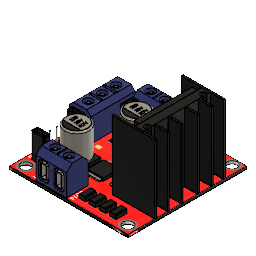
l298n (Autodesk Fusion 360 design; units mm, degrees)
Autodesk Fusion 360 part; units mm, degrees
note: some values were not read from the file. Chosen so that the rebuilt part matches the saved one: which face or edge a step refers to. Set by a fixed rule: which sketch regions a step uses.
(part 1 of 2)
sketch "Sketch2" plane through (0, 0, 0) normal (0, 1, 0) x (1, 0, 0)
  line L0 (-21.58, 21.58) -> (21.58, 21.58)
  line L1 (21.58, 21.58) -> (21.58, -21.58)
  line L2 (21.58, -21.58) -> (-21.58, -21.58)
  line L3 (-21.58, -21.58) -> (-21.58, 21.58)
  dimension "d1" = 43.16
  dimension "d2" = 43.16
extrude "Extrude1" add sketch "Sketch2" along normal blind 1 makes body 1
sketch "Sketch3" plane through (0, 1, 0) normal (0, 1, 0) x (-1, 0, 0)
  line L0 (21.58, 21.58) -> (-21.58, 21.58)
  line L1 (-21.58, 21.58) -> (-21.58, -21.58)
  line L2 (-21.58, -21.58) -> (21.58, -21.58)
  line L3 (21.58, -21.58) -> (21.58, 21.58)
  circle A0 centre (18.5683, 18.5343) radius 1.8
  circle A1 centre (-18.5859, 18.5894) radius 1.8
  circle A2 centre (18.6014, -19.35) radius 1.8
  circle A3 centre (-18.5529, -19.2949) radius 1.8
  line L4 (15.2987, 12.0305) -> (6.6207, 12.0305)
  line L5 (6.6207, 12.0305) -> (6.6207, 3.2285)
  line L6 (6.6207, 3.2285) -> (15.2987, 3.2285)
  line L7 (15.2987, 3.2285) -> (15.2987, 12.0305)
  line L8 (15.2987, 4.5307) -> (14.0438, 3.2285)
  dimension "d5" = 3.6
  dimension "d6" = 3.6
  dimension "d7" = 3.6
  dimension "d8" = 3.6
  dimension "d13" = 37.1543
  dimension "d14" = 37.1543
  measures "d5" diameter of A0
  measures "d6" diameter of A1
  measures "d7" diameter of A2
  measures "d8" diameter of A3
extrude "Extrude2" cut sketch "Sketch3" along normal blind 3 and the other way blind 2 contours A0 | A1 | A2 | A3 bodies 1
sketch "Sketch4" plane through (0, 1, 0) normal (0, 1, 0) x (-1, 0, 0)
  circle A0 centre (-18.5529, -19.2949) radius 1.8
  circle A1 centre (18.6014, -19.35) radius 1.8
  circle A2 centre (-18.5859, 18.5894) radius 1.8
  circle A3 centre (18.5683, 18.5343) radius 1.8
  line L0 (21.58, 21.58) -> (-21.58, 21.58)
  line L1 (-21.58, 21.58) -> (-21.58, -21.58)
  line L2 (-21.58, -21.58) -> (21.58, -21.58)
  line L3 (21.58, -21.58) -> (21.58, 21.58)
  line L4 (-8.5487, -11.3714) -> (-11.814, -11.3714)
  line L5 (-11.814, -11.3714) -> (-11.814, 9.6641)
  line L6 (-11.814, 9.6641) -> (-8.5487, 9.6641)
  line L7 (-8.1487, 9.2641) -> (-8.1487, -10.9714)
  arc A4 (-8.5487, -11.3714) -> (-8.1487, -10.9714) centre (-8.5487, -10.9714) ccw
  arc A5 (-8.1487, 9.2641) -> (-8.5487, 9.6641) centre (-8.5487, 9.2641) ccw
  line L8 (-13.7341, -13.1256) -> (-16.7801, -13.1256)
  line L9 (-16.7801, -13.1256) -> (-16.7801, 11.2965)
  line L10 (-16.7801, 11.2965) -> (-13.7341, 11.2965)
  line L11 (-13.7341, 11.2965) -> (-13.7341, -13.1256)
  dimension "d15" = 0.4
  dimension "d16" = 0.4
  measures "d15" radius of A4
  measures "d16" radius of A5
extrude "Extrude3" add sketch "Sketch4" along normal blind 15 contours L4 L5 L6 L7 A4 A5 bodies 1
delete_face "DeleteFace1" 7 faces at (8.2229, 11, -11.2034) (8.1487, 6, 2.5189) (8.1774, 11, 9.4127) (10.7256, 6, 9.6641) (11.814, 6, -4.3596) (9.6372, 6, -11.3714) (10.5923, 16, -4.2263) on bodies 1
sketch "Sketch5" plane through (0, 1, 0) normal (0, 1, 0) x (-1, 0, 0)
  circle A0 centre (-18.5529, -19.2949) radius 1.8
  circle A1 centre (18.6014, -19.35) radius 1.8
  circle A2 centre (-18.5859, 18.5894) radius 1.8
  circle A3 centre (18.5683, 18.5343) radius 1.8
  line L0 (-21.58, 21.58) -> (-21.58, -21.58)
  line L1 (-21.58, -21.58) -> (21.58, -21.58)
  line L2 (21.58, -21.58) -> (21.58, 21.58)
  line L3 (21.58, 21.58) -> (-21.58, 21.58)
  line L4 (-9.1628, -11.5053) -> (-11.8128, -11.5053)
  line L5 (-11.8128, -11.5053) -> (-11.8128, 9.6008)
  line L6 (-11.8128, 9.6008) -> (-9.1628, 9.6008)
  line L7 (-8.1628, 8.6008) -> (-8.1628, -10.5053)
  arc A4 (-9.1628, -11.5053) -> (-8.1628, -10.5053) centre (-9.1628, -10.5053) ccw
  arc A5 (-8.1628, 8.6008) -> (-9.1628, 9.6008) centre (-9.1628, 8.6008) ccw
  line L8 (-11.8128, -11.5053) -> (-13.7787, -11.5053)
  line L9 (-13.7787, -11.5053) -> (-13.7787, 9.5847)
  line L10 (-13.7787, 9.5847) -> (-11.8128, 9.5847)
  line L11 (-11.8128, 9.5847) -> (-11.8128, -11.5053)
  dimension "d19" = 1
  dimension "d20" = 1
  dimension "d25" = 3.65
  measures "d19" radius of A4
  measures "d20" radius of A5
  measures "d25" distance of L5 L7
extrude "Extrude8" add sketch "Sketch5" along normal blind 25 separate body contours L5 L8 L9 L10 L11 makes body 2
extrude "Extrude5" add sketch "Sketch5" along normal blind 15 separate body contours L4 L5 L6 L7 A4 A5 L11 makes body 3
sketch "Sketch6" plane through (11.8128, 0, 0) normal (1, 0, 0) x (0, 0, -1)
  line L0 (-9.6008, 1) -> (11.5053, 1)
  line L1 (11.5053, 1) -> (11.5053, 16)
  line L2 (11.5053, 16) -> (-9.6008, 16)
  line L3 (-9.6008, 16) -> (-9.6008, 1)
  circle A0 centre (-9.6008, 8.5) radius 2
  circle A1 centre (11.5053, 8.5) radius 2
  circle A2 centre (-4.6008, 8.5) radius 1
  circle A3 centre (6.5053, 8.5) radius 1
  dimension "d26" = 4
  dimension "d27" = 4
  dimension "d28" = 2
  dimension "d29" = 2
  measures "d26" diameter of A0
  measures "d27" diameter of A1
  measures "d28" diameter of A2
  measures "d29" diameter of A3
extrude "Extrude7" add sketch "Sketch6" against normal blind 4 contours A2 | A3 bodies 3
extrude "Extrude6" cut sketch "Sketch6" along normal blind 2 and the other way blind 6 contours L3 A0 | L3 A0 | L1 A1 | L1 A1 bodies 3
box "BoxPrimitive1" cut length 1.9835 width 0.2553 height -0.2 placed x (0, 1, 0) y (0, 0, -1) z (-1, 0, 0) at (7.8128, 7.5069, -6.3882) bodies 3
box "BoxPrimitive2" cut length 0.319 width 1.9733 height -0.2 placed x (0, 1, 0) y (0, 0, -1) z (-1, 0, 0) at (7.8128, 8.3724, -5.5135) bodies 3
box "BoxPrimitive3" cut length 1.9717 width 0.332 height -0.2 placed x (0, 1, 0) y (0, 0, -1) z (-1, 0, 0) at (7.8128, 7.5102, 4.7436) bodies 3
box "BoxPrimitive4" cut length 0.3057 width 1.9763 height -0.2 placed x (0, 1, 0) y (0, 0, -1) z (-1, 0, 0) at (7.8128, 8.3339, 5.587) bodies 3
box "BoxPrimitive5" add length 6.5992 width 21.1061 height 1.5 placed x (0, -1, 0) y (0, 0, 1) z (-1, 0, 0) at (11.8128, 22.5992, -11.5053) separate body makes body 4
chamfer "Chamfer1" distance 2 angle 45 1 edges at (11.0628, 22.5992, -11.5053) on bodies 4
chamfer "Chamfer2" distance 2 angle 45 1 edges at (11.0628, 22.5992, 9.6008) on bodies 4
sketch "Sketch12" plane through (10.3128, 0, 0) normal (-1, 0, 0) x (0, 0, 1)
  line L0 (9.6008, 20.5992) -> (7.6008, 22.5992)
  line L1 (7.6008, 22.5992) -> (-9.5053, 22.5992)
  line L2 (-9.5053, 22.5992) -> (-11.5053, 20.5992)
  line L3 (-11.5053, 20.5992) -> (-11.5053, 16)
  line L4 (9.6008, 16) -> (9.6008, 20.5992)
  circle A0 centre (-0.9522, 19.645) radius 1
  line L5 (-11.5053, 16) -> (9.6008, 16)
  dimension "d67" = 2
  measures "d67" diameter of A0
extrude "Extrude9" add sketch "Sketch12" along normal blind 0.5 separate body contours A0 makes body 5
box "BoxPrimitive6" cut length 1.5257 width 0.3014 height -0.5 placed x (0, 1, 0) y (0, 0, -1) z (-1, 0, 0) at (9.8128, 18.8541, -0.7916) bodies 5
box "BoxPrimitive7" cut length 0.2355 width 1.4127 height -0.5 placed x (0, 1, 0) y (0, 0, -1) z (-1, 0, 0) at (9.8128, 19.617, -0.2265) bodies 5
fillet "Fillet1" radius 0.2 1 edges at (9.8128, 19.2834, -1.8846) on bodies 5
box "BoxPrimitive8" add length 24.4221 width 3.046 height 25 placed x (0, 0, 1) y (1, 0, 0) z (0, 1, 0) at (13.7341, 1, -13.1256) separate body makes body 6
cylinder "CylinderPrimitive1" cut diameter 2 height -25 placed x (1, 0, 0) y (0, 0, -1) z (0, 1, 0) at (16.0686, 26, -11.2277) bodies 6
cylinder "CylinderPrimitive2" cut diameter 2 height -25 placed x (1, 0, 0) y (0, 0, -1) z (0, 1, 0) at (16.0862, 26, 9.0521) bodies 6
box "BoxPrimitive9" add length 0.6958 width 15.4001 height 25 placed x (0, 0, 1) y (1, 0, 0) z (0, 1, 0) at (6.1799, 1, 11.1734) separate body makes body 7
copy_body "CopyPasteBodies1" bodies 7 makes body 8
move_body "Move1" bodies 8 to x (1, 0, 0) y (0, 1, 0) z (0, 0, 1) at (0, 0, -25)
box "BoxPrimitive20" add length 0.9521 width 4.9337 height 0.5 placed x (0, 0, 1) y (1, 0, 0) z (0, 1, 0) at (-4.9818, 1, 9.3224) separate body makes body 9
box "BoxPrimitive10" add length 0.6636 width 4.7999 height 25 placed x (0, 0, -1) y (-1, 0, 0) z (0, 1, 0) at (21.58, 1, 7.2397) separate body makes body 10
copy_body "CopyPasteBodies2" bodies 10 makes body 11
move_body "Move2" bodies 11 to x (1, 0, 0) y (0, 1, 0) z (0, 0, 1) at (0, 0, -5)
copy_body "CopyPasteBodies3" bodies 11 makes body 12
move_body "Move3" bodies 12 to x (1, 0, 0) y (0, 1, 0) z (0, 0, 1) at (0, 0, -6)
copy_body "CopyPasteBodies4" bodies 12 makes body 13
move_body "Move4" bodies 13 to x (1, 0, 0) y (0, 1, 0) z (0, 0, 1) at (0, 0, -5)
box "BoxPrimitive11" add length 8.802 width 8.678 height 1 placed x (0, 0, 1) y (1, 0, 0) z (0, 1, 0) at (-15.2987, 1, 3.2285) separate body makes body 14
copy_body "CopyPasteBodies5" bodies 14 makes body 15
move_body "Move5" bodies 15 to x (1, 0, 0) y (0, 1, 0) z (0, 0, 1) at (7.2382, 0, -14.5913)
sketch "Sketch23" plane through (0, 2, 0) normal (0, 1, 0) x (-1, 0, 0)
  line L0 (15.2987, 12.0305) -> (6.6207, 12.0305)
  line L1 (6.6207, 12.0305) -> (6.6207, 3.2285)
  line L2 (6.6207, 3.2285) -> (15.2987, 3.2285)
  line L3 (15.2987, 3.2285) -> (15.2987, 12.0305)
  line L4 (15.2987, 3.2285) -> (6.6207, 12.0305) construction
  line L5 (6.6207, 3.2285) -> (15.2987, 12.0305) construction
cylinder "CylinderPrimitive3" add diameter 8.678 height 11 placed x (1, 0, 0) y (0, 0, -1) z (0, 1, 0) at (-10.9597, 2, 7.6295) separate body makes body 16
fillet "Fillet2" radius 1 1 edges at (-15.005, 2, 6.0605) on bodies 16
fillet "Fillet3" radius 0.5 1 edges at (-15.005, 13, 9.1986) on bodies 16
sketch "Sketch24" plane through (0, 13, 0) normal (0, 1, 0) x (-1, 0, 0)
  circle A0 centre (10.9597, 7.6295) radius 3.839
  line L0 (14.3816, 9.3698) -> (7.5378, 9.3698)
extrude "Extrude11" add sketch "Sketch24" along normal blind 0.1 contours A0 L0 picked at (9.791, 7.9606) bodies 16
extrude "Extrude10" add sketch "Sketch24" along normal blind 0.1 separate body contours A0 L0 picked at (10.272, 9.961) makes body 17
fillet "Fillet4" radius 0.1 1 edges at (-10.9597, 13.1, 11.4685) on bodies 17
fillet "Fillet5" radius 0.1 1 edges at (-10.9597, 13.1, 3.7905) on bodies 16
sketch "Sketch25" plane through (0, 13.1, 0) normal (0, 1, 0) x (-1, 0, 0)
  arc A0 (7.6504, 9.3698) -> (14.269, 9.3698) centre (10.9597, 7.6295) ccw
  line L0 (14.269, 9.3698) -> (7.6504, 9.3698)
  line L1 (12.3518, 7.4819) -> (12.1607, 7.4819)
  line L2 (12.1607, 7.4819) -> (12.1607, 8.2033)
  spline S0 degree 3 poles (12.1607, 8.2033) (12.1965, 8.1973) (12.2689, 8.1853) (12.3335, 8.1505) (12.3661, 8.133) knots 0 0 0 0 0.010813 0.021847 0.021847 0.021847 0.021847
  spline S1 degree 3 poles (12.3661, 8.133) (12.4046, 8.1049) (12.4981, 8.0365) (12.5771, 7.9515) (12.6236, 7.9015) knots 0 0 0 0 0.014262 0.034686 0.034686 0.034686 0.034686
  spline S2 degree 3 poles (12.6236, 7.9015) (12.6589, 7.8631) (12.7142, 7.8028) (12.7767, 7.75) (12.7993, 7.7309) knots 0 0 0 0 0.01563 0.024519 0.024519 0.024519 0.024519
  spline S3 degree 3 poles (12.7993, 7.7309) (12.8199, 7.7185) (12.8588, 7.695) (12.904, 7.6905) (12.9253, 7.6884) knots 0 0 0 0 0.007091 0.013443 0.013443 0.013443 0.013443
  spline S4 degree 3 poles (12.9253, 7.6884) (12.9464, 7.6894) (12.9855, 7.6913) (13.0167, 7.7146) (13.0312, 7.7254) knots 0 0 0 0 0.006158 0.01144 0.01144 0.01144 0.01144
  spline S5 degree 3 poles (13.0312, 7.7254) (13.0419, 7.7395) (13.0649, 7.7695) (13.067, 7.8074) (13.0681, 7.8276) knots 0 0 0 0 0.005205 0.011091 0.011091 0.011091 0.011091
  spline S6 degree 3 poles (13.0681, 7.8276) (13.0669, 7.8476) (13.0644, 7.8859) (13.0406, 7.9158) (13.0293, 7.9301) knots 0 0 0 0 0.005867 0.0112 0.0112 0.0112 0.0112
  spline S7 degree 3 poles (13.0293, 7.9301) (13.0126, 7.9415) (12.974, 7.9679) (12.9271, 7.9718) (12.9004, 7.974) knots 0 0 0 0 0.005973 0.013825 0.013825 0.013825 0.013825
  line L3 (12.9004, 7.974) -> (12.9209, 8.1791)
  spline S8 degree 3 poles (12.9209, 8.1791) (12.9721, 8.1715) (13.0655, 8.1577) (13.1339, 8.0933) (13.1648, 8.0641) knots 0 0 0 0 0.015078 0.027543 0.027543 0.027543 0.027543
  spline S9 degree 3 poles (13.1648, 8.0641) (13.1864, 8.0288) (13.2317, 7.9548) (13.2363, 7.8679) (13.2388, 7.8224) knots 0 0 0 0 0.01221 0.025631 0.025631 0.025631 0.025631
  spline S10 degree 3 poles (13.2388, 7.8224) (13.2363, 7.7735) (13.2316, 7.6817) (13.1781, 7.6074) (13.1531, 7.5727) knots 0 0 0 0 0.014351 0.026906 0.026906 0.026906 0.026906
  spline S11 degree 3 poles (13.1531, 7.5727) (13.1227, 7.5462) (13.0615, 7.4929) (12.9806, 7.4856) (12.94, 7.4819) knots 0 0 0 0 0.011782 0.0237 0.0237 0.0237 0.0237
  spline S12 degree 3 poles (12.94, 7.4819) (12.9162, 7.4829) (12.8689, 7.485) (12.8241, 7.5003) (12.8019, 7.5079) knots 0 0 0 0 0.007107 0.014113 0.014113 0.014113 0.014113
  spline S13 degree 3 poles (12.8019, 7.5079) (12.7791, 7.5183) (12.7303, 7.5408) (12.6874, 7.5731) (12.6646, 7.5903) knots 0 0 0 0 0.007505 0.016056 0.016056 0.016056 0.016056
  spline S14 degree 3 poles (12.6646, 7.5903) (12.645, 7.6074) (12.5967, 7.6497) (12.5534, 7.697) (12.5276, 7.725) knots 0 0 0 0 0.007818 0.019227 0.019227 0.019227 0.019227
  spline S15 degree 3 poles (12.5276, 7.725) (12.5032, 7.7519) (12.4647, 7.7941) (12.4238, 7.8339) (12.409, 7.8484) knots 0 0 0 0 0.010889 0.017123 0.017123 0.017123 0.017123
  spline S16 degree 3 poles (12.409, 7.8484) (12.3995, 7.8565) (12.3815, 7.872) (12.3614, 7.8846) (12.3518, 7.8905) knots 0 0 0 0 0.003729 0.007106 0.007106 0.007106 0.007106
  line L4 (12.3518, 7.8905) -> (12.3518, 7.4819)
  line L5 (12.3518, 6.6476) -> (12.1607, 6.6476)
  line L6 (12.1607, 6.6476) -> (12.1607, 7.3691)
  spline S17 degree 3 poles (12.1607, 7.3691) (12.1965, 7.3631) (12.2689, 7.3511) (12.3335, 7.3163) (12.3661, 7.2987) knots 0 0 0 0 0.010813 0.021847 0.021847 0.021847 0.021847
  spline S18 degree 3 poles (12.3661, 7.2987) (12.4046, 7.2706) (12.4981, 7.2022) (12.5771, 7.1173) (12.6236, 7.0673) knots 0 0 0 0 0.014262 0.034686 0.034686 0.034686 0.034686
  spline S19 degree 3 poles (12.6236, 7.0673) (12.6589, 7.0289) (12.7142, 6.9686) (12.7767, 6.9158) (12.7993, 6.8967) knots 0 0 0 0 0.01563 0.024519 0.024519 0.024519 0.024519
  spline S20 degree 3 poles (12.7993, 6.8967) (12.8199, 6.8843) (12.8588, 6.8608) (12.904, 6.8563) (12.9253, 6.8542) knots 0 0 0 0 0.007091 0.013443 0.013443 0.013443 0.013443
  spline S21 degree 3 poles (12.9253, 6.8542) (12.9464, 6.8552) (12.9855, 6.8571) (13.0167, 6.8804) (13.0312, 6.8912) knots 0 0 0 0 0.006158 0.01144 0.01144 0.01144 0.01144
  spline S22 degree 3 poles (13.0312, 6.8912) (13.0419, 6.9053) (13.0649, 6.9353) (13.067, 6.9732) (13.0681, 6.9933) knots 0 0 0 0 0.005205 0.011091 0.011091 0.011091 0.011091
  spline S23 degree 3 poles (13.0681, 6.9933) (13.0669, 7.0134) (13.0644, 7.0516) (13.0406, 7.0816) (13.0293, 7.0959) knots 0 0 0 0 0.005867 0.0112 0.0112 0.0112 0.0112
  spline S24 degree 3 poles (13.0293, 7.0959) (13.0126, 7.1073) (12.974, 7.1337) (12.9271, 7.1376) (12.9004, 7.1398) knots 0 0 0 0 0.005973 0.013825 0.013825 0.013825 0.013825
  line L7 (12.9004, 7.1398) -> (12.9209, 7.3449)
  spline S25 degree 3 poles (12.9209, 7.3449) (12.9721, 7.3373) (13.0655, 7.3235) (13.1339, 7.259) (13.1648, 7.2299) knots 0 0 0 0 0.015078 0.027543 0.027543 0.027543 0.027543
  spline S26 degree 3 poles (13.1648, 7.2299) (13.1864, 7.1946) (13.2317, 7.1205) (13.2363, 7.0337) (13.2388, 6.9882) knots 0 0 0 0 0.01221 0.025631 0.025631 0.025631 0.025631
  spline S27 degree 3 poles (13.2388, 6.9882) (13.2363, 6.9392) (13.2316, 6.8475) (13.1781, 6.7731) (13.1531, 6.7384) knots 0 0 0 0 0.014351 0.026906 0.026906 0.026906 0.026906
  spline S28 degree 3 poles (13.1531, 6.7384) (13.1227, 6.712) (13.0615, 6.6587) (12.9806, 6.6513) (12.94, 6.6476) knots 0 0 0 0 0.011782 0.0237 0.0237 0.0237 0.0237
  spline S29 degree 3 poles (12.94, 6.6476) (12.9162, 6.6487) (12.8689, 6.6508) (12.8241, 6.666) (12.8019, 6.6736) knots 0 0 0 0 0.007107 0.014113 0.014113 0.014113 0.014113
  spline S30 degree 3 poles (12.8019, 6.6736) (12.7791, 6.6841) (12.7303, 6.7065) (12.6874, 6.7388) (12.6646, 6.756) knots 0 0 0 0 0.007505 0.016056 0.016056 0.016056 0.016056
  spline S31 degree 3 poles (12.6646, 6.756) (12.645, 6.7732) (12.5967, 6.8155) (12.5534, 6.8627) (12.5276, 6.8908) knots 0 0 0 0 0.007818 0.019227 0.019227 0.019227 0.019227
  spline S32 degree 3 poles (12.5276, 6.8908) (12.5032, 6.9176) (12.4647, 6.9598) (12.4238, 6.9997) (12.409, 7.0142) knots 0 0 0 0 0.010889 0.017123 0.017123 0.017123 0.017123
  spline S33 degree 3 poles (12.409, 7.0142) (12.3995, 7.0223) (12.3815, 7.0378) (12.3614, 7.0503) (12.3518, 7.0563) knots 0 0 0 0 0.003729 0.007106 0.007106 0.007106 0.007106
  line L8 (12.3518, 7.0563) -> (12.3518, 6.6476)
  spline S34 degree 3 poles (13.2388, 6.1606) (13.2347, 6.1118) (13.2267, 6.017) (13.1599, 5.9495) (13.1275, 5.9167) knots 0 0 0 0 0.014174 0.027582 0.027582 0.027582 0.027582
  spline S35 degree 3 poles (13.1275, 5.9167) (13.0702, 5.8863) (12.9343, 5.8143) (12.7797, 5.8128) (12.6902, 5.8119) knots 0 0 0 0 0.019203 0.045536 0.045536 0.045536 0.045536
  spline S36 degree 3 poles (12.6902, 5.8119) (12.6008, 5.8129) (12.4459, 5.8146) (12.3098, 5.8868) (12.2522, 5.9174) knots 0 0 0 0 0.026317 0.045626 0.045626 0.045626 0.045626
  spline S37 degree 3 poles (12.2522, 5.9174) (12.2202, 5.9501) (12.1541, 6.0175) (12.1463, 6.1119) (12.1424, 6.1606) knots 0 0 0 0 0.013298 0.027446 0.027446 0.027446 0.027446
  spline S38 degree 3 poles (12.1424, 6.1606) (12.1473, 6.2102) (12.1571, 6.309) (12.2277, 6.3786) (12.2628, 6.4133) knots 0 0 0 0 0.014471 0.028795 0.028795 0.028795 0.028795
  spline S39 degree 3 poles (12.2628, 6.4133) (12.3178, 6.441) (12.4519, 6.5088) (12.6031, 6.5091) (12.6924, 6.5092) knots 0 0 0 0 0.018243 0.044545 0.044545 0.044545 0.044545
  spline S40 degree 3 poles (12.6924, 6.5092) (12.7814, 6.5082) (12.9359, 6.5065) (13.0715, 6.4343) (13.1289, 6.4037) knots 0 0 0 0 0.026207 0.045483 0.045483 0.045483 0.045483
  spline S41 degree 3 poles (13.1289, 6.4037) (13.161, 6.371) (13.2271, 6.3036) (13.2348, 6.2092) (13.2388, 6.1606) knots 0 0 0 0 0.013298 0.027446 0.027446 0.027446 0.027446
  spline S42 degree 3 poles (13.0681, 6.1606) (13.0671, 6.1727) (13.0651, 6.197) (13.0513, 6.2171) (13.0443, 6.2272) knots 0 0 0 0 0.003584 0.007188 0.007188 0.007188 0.007188
  spline S43 degree 3 poles (13.0443, 6.2272) (13.0337, 6.2367) (13.0091, 6.2587) (12.9772, 6.2676) (12.959, 6.2726) knots 0 0 0 0 0.00422 0.009779 0.009779 0.009779 0.009779
  spline S44 degree 3 poles (12.959, 6.2726) (12.9234, 6.2788) (12.8345, 6.2941) (12.7443, 6.2939) (12.6902, 6.2939) knots 0 0 0 0 0.010829 0.027006 0.027006 0.027006 0.027006
  spline S45 degree 3 poles (12.6902, 6.2939) (12.6369, 6.2941) (12.5498, 6.2944) (12.4639, 6.2803) (12.4306, 6.2748) knots 0 0 0 0 0.015946 0.026073 0.026073 0.026073 0.026073
  spline S46 degree 3 poles (12.4306, 6.2748) (12.4101, 6.2692) (12.3752, 6.2597) (12.3478, 6.2364) (12.3365, 6.2269) knots 0 0 0 0 0.006268 0.010675 0.010675 0.010675 0.010675
  spline S47 degree 3 poles (12.3365, 6.2269) (12.3296, 6.2169) (12.3159, 6.1968) (12.314, 6.1727) (12.313, 6.1606) knots 0 0 0 0 0.003567 0.00714 0.00714 0.00714 0.00714
  spline S48 degree 3 poles (12.313, 6.1606) (12.314, 6.1484) (12.316, 6.1241) (12.3299, 6.104) (12.3368, 6.0939) knots 0 0 0 0 0.003584 0.007188 0.007188 0.007188 0.007188
  spline S49 degree 3 poles (12.3368, 6.0939) (12.3474, 6.0844) (12.3721, 6.0625) (12.404, 6.0536) (12.4222, 6.0485) knots 0 0 0 0 0.00422 0.009779 0.009779 0.009779 0.009779
  spline S50 degree 3 poles (12.4222, 6.0485) (12.4576, 6.0424) (12.5462, 6.027) (12.6362, 6.0272) (12.6902, 6.0273) knots 0 0 0 0 0.010775 0.026934 0.026934 0.026934 0.026934
  spline S51 degree 3 poles (12.6902, 6.0273) (12.7435, 6.027) (12.8306, 6.0267) (12.9165, 6.0408) (12.9499, 6.0463) knots 0 0 0 0 0.015946 0.026073 0.026073 0.026073 0.026073
  spline S52 degree 3 poles (12.9499, 6.0463) (12.9704, 6.0519) (13.0053, 6.0615) (13.0329, 6.0847) (13.0443, 6.0943) knots 0 0 0 0 0.006276 0.010706 0.010706 0.010706 0.010706
  spline S53 degree 3 poles (13.0443, 6.0943) (13.0513, 6.1043) (13.0652, 6.1242) (13.0672, 6.1485) (13.0681, 6.1606) knots 0 0 0 0 0.00358 0.007155 0.007155 0.007155 0.007155
  line L9 (10.5927, 8.3502) -> (10.6103, 8.2184)
  spline S54 degree 3 poles (10.6103, 8.2184) (10.5768, 8.2108) (10.5169, 8.1972) (10.4697, 8.1583) (10.4488, 8.1411) knots 0 0 0 0 0.010117 0.018122 0.018122 0.018122 0.018122
  spline S55 degree 3 poles (10.4488, 8.1411) (10.4344, 8.1217) (10.405, 8.0822) (10.4013, 8.0332) (10.3993, 8.0082) knots 0 0 0 0 0.007097 0.014444 0.014444 0.014444 0.014444
  spline S56 degree 3 poles (10.3993, 8.0082) (10.402, 7.9785) (10.4072, 7.9194) (10.445, 7.8738) (10.4638, 7.8511) knots 0 0 0 0 0.008729 0.017344 0.017344 0.017344 0.017344
  spline S57 degree 3 poles (10.4638, 7.8511) (10.4868, 7.8324) (10.5333, 7.7945) (10.5931, 7.7895) (10.6235, 7.787) knots 0 0 0 0 0.008669 0.017567 0.017567 0.017567 0.017567
  spline S58 degree 3 poles (10.6235, 7.787) (10.6522, 7.7892) (10.7083, 7.7936) (10.7519, 7.829) (10.7732, 7.8463) knots 0 0 0 0 0.008417 0.016454 0.016454 0.016454 0.016454
  spline S59 degree 3 poles (10.7732, 7.8463) (10.7904, 7.8678) (10.8257, 7.9119) (10.83, 7.9683) (10.8322, 7.9972) knots 0 0 0 0 0.00806 0.016538 0.016538 0.016538 0.016538
  spline S60 degree 3 poles (10.8322, 7.9972) (10.8314, 8.0112) (10.8295, 8.0427) (10.8218, 8.0733) (10.8176, 8.0902) knots 0 0 0 0 0.004209 0.009435 0.009435 0.009435 0.009435
  line L10 (10.8176, 8.0902) -> (10.9333, 8.0756)
  spline S61 degree 3 poles (10.9333, 8.0756) (10.9329, 8.0716) (10.9321, 8.0645) (10.9319, 8.0574) (10.9318, 8.0543) knots 0 0 0 0 0.001195 0.00213 0.00213 0.00213 0.00213
  spline S62 degree 3 poles (10.9318, 8.0543) (10.9336, 8.0271) (10.937, 7.9733) (10.9629, 7.926) (10.9758, 7.9027) knots 0 0 0 0 0.008077 0.015958 0.015958 0.015958 0.015958
  spline S63 degree 3 poles (10.9758, 7.9027) (10.9929, 7.8831) (11.0287, 7.8422) (11.083, 7.8377) (11.1113, 7.8353) knots 0 0 0 0 0.007532 0.015673 0.015673 0.015673 0.015673
  spline S64 degree 3 poles (11.1113, 7.8353) (11.1342, 7.8372) (11.1795, 7.841) (11.2143, 7.8701) (11.2314, 7.8844) knots 0 0 0 0 0.006741 0.013262 0.013262 0.013262 0.013262
  spline S65 degree 3 poles (11.2314, 7.8844) (11.2453, 7.9024) (11.274, 7.9397) (11.2773, 7.9867) (11.279, 8.0111) knots 0 0 0 0 0.006659 0.013809 0.013809 0.013809 0.013809
  spline S66 degree 3 poles (11.279, 8.0111) (11.2772, 8.0355) (11.2736, 8.083) (11.2447, 8.1208) (11.2306, 8.1393) knots 0 0 0 0 0.007152 0.013965 0.013965 0.013965 0.013965
  spline S67 degree 3 poles (11.2306, 8.1393) (11.2113, 8.155) (11.1689, 8.1895) (11.115, 8.1997) (11.0856, 8.2052) knots 0 0 0 0 0.007365 0.016153 0.016153 0.016153 0.016153
  line L11 (11.0856, 8.2052) -> (11.1091, 8.337)
  spline S68 degree 3 poles (11.1091, 8.337) (11.1501, 8.3272) (11.2283, 8.3084) (11.2867, 8.2534) (11.3145, 8.2272) knots 0 0 0 0 0.012412 0.02366 0.02366 0.02366 0.02366
  spline S69 degree 3 poles (11.3145, 8.2272) (11.3357, 8.1962) (11.3798, 8.132) (11.3848, 8.0543) (11.3874, 8.014) knots 0 0 0 0 0.011058 0.0229 0.0229 0.0229 0.0229
  spline S70 degree 3 poles (11.3874, 8.014) (11.3859, 7.9855) (11.383, 7.9293) (11.3607, 7.8776) (11.3497, 7.8522) knots 0 0 0 0 0.008494 0.01674 0.01674 0.01674 0.01674
  spline S71 degree 3 poles (11.3497, 7.8522) (11.3362, 7.8291) (11.3099, 7.7841) (11.2675, 7.7538) (11.2468, 7.739) knots 0 0 0 0 0.007905 0.015451 0.015451 0.015451 0.015451
  spline S72 degree 3 poles (11.2468, 7.739) (11.2248, 7.7276) (11.1814, 7.705) (11.1325, 7.7015) (11.1083, 7.6998) knots 0 0 0 0 0.007335 0.014524 0.014524 0.014524 0.014524
  spline S73 degree 3 poles (11.1083, 7.6998) (11.0857, 7.7014) (11.0407, 7.7044) (11.0012, 7.7263) (10.9816, 7.7372) knots 0 0 0 0 0.006712 0.013356 0.013356 0.013356 0.013356
  spline S74 degree 3 poles (10.9816, 7.7372) (10.9633, 7.7516) (10.9251, 7.7819) (10.9025, 7.8252) (10.8908, 7.8478) knots 0 0 0 0 0.00691 0.014456 0.014456 0.014456 0.014456
  spline S75 degree 3 poles (10.8908, 7.8478) (10.8819, 7.8181) (10.8646, 7.7606) (10.8208, 7.7197) (10.7996, 7.6998) knots 0 0 0 0 0.009109 0.017658 0.017658 0.017658 0.017658
  spline S76 degree 3 poles (10.7996, 7.6998) (10.7743, 7.6845) (10.7212, 7.6522) (10.659, 7.6488) (10.6264, 7.6471) knots 0 0 0 0 0.008738 0.018359 0.018359 0.018359 0.018359
  spline S77 degree 3 poles (10.6264, 7.6471) (10.5813, 7.6514) (10.4908, 7.66) (10.4223, 7.7197) (10.388, 7.7496) knots 0 0 0 0 0.013242 0.02654 0.02654 0.02654 0.02654
  spline S78 degree 3 poles (10.388, 7.7496) (10.3595, 7.7868) (10.3008, 7.8632) (10.2938, 7.9594) (10.2902, 8.0089) knots 0 0 0 0 0.013731 0.028257 0.028257 0.028257 0.028257
  spline S79 degree 3 poles (10.2902, 8.0089) (10.2932, 8.0535) (10.2991, 8.1399) (10.3499, 8.2098) (10.3744, 8.2437) knots 0 0 0 0 0.013107 0.025393 0.025393 0.025393 0.025393
  spline S80 degree 3 poles (10.3744, 8.2437) (10.405, 8.2715) (10.4673, 8.3282) (10.5504, 8.3428) (10.5927, 8.3502) knots 0 0 0 0 0.012135 0.024739 0.024739 0.024739 0.024739
  line L12 (10.5905, 7.5167) -> (10.6022, 7.3783)
  spline S81 degree 3 poles (10.6022, 7.3783) (10.5715, 7.3724) (10.5146, 7.3613) (10.4705, 7.324) (10.4502, 7.3069) knots 0 0 0 0 0.009214 0.017043 0.017043 0.017043 0.017043
  spline S82 degree 3 poles (10.4502, 7.3069) (10.4354, 7.2871) (10.4053, 7.247) (10.4014, 7.1971) (10.3993, 7.1718) knots 0 0 0 0 0.007264 0.014707 0.014707 0.014707 0.014707
  spline S83 degree 3 poles (10.3993, 7.1718) (10.4024, 7.1412) (10.4086, 7.0796) (10.4502, 7.0337) (10.4711, 7.0106) knots 0 0 0 0 0.00897 0.01806 0.01806 0.01806 0.01806
  spline S84 degree 3 poles (10.4711, 7.0106) (10.498, 6.9914) (10.5548, 6.9508) (10.6247, 6.9468) (10.6615, 6.9447) knots 0 0 0 0 0.009703 0.020523 0.020523 0.020523 0.020523
  spline S85 degree 3 poles (10.6615, 6.9447) (10.6964, 6.9467) (10.7622, 6.9503) (10.8148, 6.9896) (10.8395, 7.0081) knots 0 0 0 0 0.010213 0.019268 0.019268 0.019268 0.019268
  spline S86 degree 3 poles (10.8395, 7.0081) (10.8585, 7.0314) (10.8979, 7.0796) (10.9024, 7.1418) (10.9047, 7.174) knots 0 0 0 0 0.008798 0.018215 0.018215 0.018215 0.018215
  spline S87 degree 3 poles (10.9047, 7.174) (10.9036, 7.1945) (10.9014, 7.2347) (10.8842, 7.2711) (10.8758, 7.2889) knots 0 0 0 0 0.006104 0.011959 0.011959 0.011959 0.011959
  spline S88 degree 3 poles (10.8758, 7.2889) (10.8656, 7.305) (10.8456, 7.3366) (10.8155, 7.3587) (10.8007, 7.3695) knots 0 0 0 0 0.005657 0.011098 0.011098 0.011098 0.011098
  line L13 (10.8007, 7.3695) -> (10.8168, 7.4933)
  line L14 (10.8168, 7.4933) -> (11.3683, 7.3893)
  line L15 (11.3683, 7.3893) -> (11.3683, 6.8554)
  line L16 (11.3683, 6.8554) -> (11.2424, 6.8554)
  line L17 (11.2424, 6.8554) -> (11.2424, 7.2838)
  line L18 (11.2424, 7.2838) -> (10.9538, 7.3417)
  spline S89 degree 3 poles (10.9538, 7.3417) (10.9734, 7.3096) (11.0117, 7.2471) (11.0181, 7.1742) (11.0212, 7.1388) knots 0 0 0 0 0.011121 0.021639 0.021639 0.021639 0.021639
  spline S90 degree 3 poles (11.0212, 7.1388) (11.0172, 7.0939) (11.0094, 7.0046) (10.9522, 6.9357) (10.9238, 6.9015) knots 0 0 0 0 0.013191 0.026202 0.026202 0.026202 0.026202
  spline S91 degree 3 poles (10.9238, 6.9015) (10.8882, 6.8733) (10.8149, 6.8151) (10.7214, 6.8083) (10.6733, 6.8048) knots 0 0 0 0 0.013286 0.02741 0.02741 0.02741 0.02741
  spline S92 degree 3 poles (10.6733, 6.8048) (10.6267, 6.8081) (10.5352, 6.8145) (10.4588, 6.865) (10.4213, 6.8898) knots 0 0 0 0 0.013751 0.026994 0.026994 0.026994 0.026994
  spline S93 degree 3 poles (10.4213, 6.8898) (10.3833, 6.9279) (10.3056, 7.0059) (10.2959, 7.1157) (10.2909, 7.1718) knots 0 0 0 0 0.015645 0.031959 0.031959 0.031959 0.031959
  spline S94 degree 3 poles (10.2909, 7.1718) (10.2937, 7.2176) (10.2989, 7.3051) (10.3491, 7.3767) (10.373, 7.4109) knots 0 0 0 0 0.01346 0.025725 0.025725 0.025725 0.025725
  spline S95 degree 3 poles (10.373, 7.4109) (10.4031, 7.4385) (10.465, 7.4953) (10.5479, 7.5095) (10.5905, 7.5167) knots 0 0 0 0 0.011999 0.024652 0.024652 0.024652 0.024652
  line L19 (10.3093, 6.3222) -> (11.383, 6.7382)
  line L20 (11.383, 6.7382) -> (11.383, 6.5844)
  line L21 (11.383, 6.5844) -> (10.603, 6.3053)
  spline S96 degree 3 poles (10.603, 6.3053) (10.5728, 6.2947) (10.5147, 6.2743) (10.4556, 6.2571) (10.4272, 6.2489) knots 0 0 0 0 0.009595 0.018464 0.018464 0.018464 0.018464
  spline S97 degree 3 poles (10.4272, 6.2489) (10.4566, 6.2402) (10.5158, 6.2228) (10.5738, 6.2017) (10.603, 6.191) knots 0 0 0 0 0.009192 0.01851 0.01851 0.01851 0.01851
  line L22 (10.603, 6.191) -> (11.383, 5.901)
  line L23 (11.383, 5.901) -> (11.383, 5.756)
  line L24 (11.383, 5.756) -> (10.3093, 6.1764)
  line L25 (10.3093, 6.1764) -> (10.3093, 6.3222)
  line L26 (8.5571, 8.4972) -> (9.6308, 8.4972)
  line L27 (9.6308, 8.4972) -> (9.6308, 8.0211)
  spline S98 degree 3 poles (9.6308, 8.0211) (9.6305, 7.9787) (9.6299, 7.9046) (9.6103, 7.8333) (9.6019, 7.8028) knots 0 0 0 0 0.012655 0.022099 0.022099 0.022099 0.022099
  spline S99 degree 3 poles (9.6019, 7.8028) (9.5902, 7.779) (9.5663, 7.7306) (9.5222, 7.6994) (9.4997, 7.6834) knots 0 0 0 0 0.007821 0.015937 0.015937 0.015937 0.015937
  spline S100 degree 3 poles (9.4997, 7.6834) (9.4745, 7.6704) (9.4237, 7.6441) (9.3666, 7.6406) (9.3378, 7.6388) knots 0 0 0 0 0.008406 0.016957 0.016957 0.016957 0.016957
  spline S101 degree 3 poles (9.3378, 7.6388) (9.3015, 7.6416) (9.2299, 7.6473) (9.1731, 7.6912) (9.1452, 7.7127) knots 0 0 0 0 0.01069 0.021037 0.021037 0.021037 0.021037
  spline S102 degree 3 poles (9.1452, 7.7127) (9.1212, 7.7429) (9.0679, 7.8099) (9.0535, 7.8947) (9.0456, 7.9413) knots 0 0 0 0 0.011386 0.025288 0.025288 0.025288 0.025288
  spline S103 degree 3 poles (9.0456, 7.9413) (9.0372, 7.9243) (9.0222, 7.894) (9.0014, 7.8673) (8.9921, 7.8556) knots 0 0 0 0 0.005645 0.010124 0.010124 0.010124 0.010124
  spline S104 degree 3 poles (8.9921, 7.8556) (8.9713, 7.8347) (8.9274, 7.7908) (8.8762, 7.7559) (8.8493, 7.7376) knots 0 0 0 0 0.008834 0.018558 0.018558 0.018558 0.018558
  line L28 (8.8493, 7.7376) -> (8.5571, 7.5509)
  line L29 (8.5571, 7.5509) -> (8.5571, 7.7296)
  line L30 (8.5571, 7.7296) -> (8.7805, 7.8717)
  spline S105 degree 3 poles (8.7805, 7.8717) (8.8091, 7.8902) (8.8595, 7.9229) (8.9077, 7.9588) (8.9284, 7.9742) knots 0 0 0 0 0.010248 0.018005 0.018005 0.018005 0.018005
  spline S106 degree 3 poles (8.9284, 7.9742) (8.9436, 7.9863) (8.9702, 8.0077) (8.9911, 8.0347) (9.0002, 8.0464) knots 0 0 0 0 0.005794 0.010208 0.010208 0.010208 0.010208
  spline S107 degree 3 poles (9.0002, 8.0464) (9.0065, 8.0569) (9.0187, 8.0773) (9.0255, 8.1001) (9.0287, 8.1112) knots 0 0 0 0 0.003654 0.007108 0.007108 0.007108 0.007108
  spline S108 degree 3 poles (9.0287, 8.1112) (9.0302, 8.1218) (9.0339, 8.148) (9.0339, 8.1745) (9.0339, 8.1903) knots 0 0 0 0 0.003209 0.007935 0.007935 0.007935 0.007935
  line L31 (9.0339, 8.1903) -> (9.0339, 8.3551)
  line L32 (9.0339, 8.3551) -> (8.5571, 8.3551)
  line L33 (8.5571, 8.3551) -> (8.5571, 8.4972)
  line L34 (9.1569, 8.3551) -> (9.1569, 8.0497)
  spline S109 degree 3 poles (9.1569, 8.0497) (9.1572, 8.0205) (9.1578, 7.9689) (9.1712, 7.919) (9.1771, 7.8973) knots 0 0 0 0 0.008694 0.015421 0.015421 0.015421 0.015421
  spline S110 degree 3 poles (9.1771, 7.8973) (9.1846, 7.8802) (9.1992, 7.847) (9.2277, 7.8247) (9.2415, 7.8138) knots 0 0 0 0 0.005498 0.010694 0.010694 0.010694 0.010694
  spline S111 degree 3 poles (9.2415, 7.8138) (9.2566, 7.8055) (9.2866, 7.7889) (9.3208, 7.7865) (9.3378, 7.7853) knots 0 0 0 0 0.005096 0.010154 0.010154 0.010154 0.010154
  spline S112 degree 3 poles (9.3378, 7.7853) (9.362, 7.7875) (9.41, 7.7919) (9.4455, 7.8244) (9.4631, 7.8406) knots 0 0 0 0 0.007076 0.014032 0.014032 0.014032 0.014032
  spline S113 degree 3 poles (9.4631, 7.8406) (9.4773, 7.8637) (9.5101, 7.9169) (9.5114, 7.9798) (9.5121, 8.0152) knots 0 0 0 0 0.008026 0.018434 0.018434 0.018434 0.018434
  line L35 (9.5121, 8.0152) -> (9.5121, 8.3551)
  line L36 (9.5121, 8.3551) -> (9.1569, 8.3551)
  line L37 (8.5571, 7.17) -> (9.5041, 7.17)
  line L38 (9.5041, 7.17) -> (9.5041, 7.5238)
  line L39 (9.5041, 7.5238) -> (9.6308, 7.5238)
  line L40 (9.6308, 7.5238) -> (9.6308, 6.6727)
  line L41 (9.6308, 6.6727) -> (9.5041, 6.6727)
  line L42 (9.5041, 6.6727) -> (9.5041, 7.0279)
  line L43 (9.5041, 7.0279) -> (8.5571, 7.0279)
  line L44 (8.5571, 7.0279) -> (8.5571, 7.17)
  line L45 (8.5571, 6.2201) -> (9.6308, 6.6361)
  line L46 (9.6308, 6.6361) -> (9.6308, 6.4823)
  line L47 (9.6308, 6.4823) -> (8.8508, 6.2032)
  spline S114 degree 3 poles (8.8508, 6.2032) (8.8206, 6.1926) (8.7625, 6.1722) (8.7034, 6.1551) (8.675, 6.1468) knots 0 0 0 0 0.009595 0.018464 0.018464 0.018464 0.018464
  spline S115 degree 3 poles (8.675, 6.1468) (8.7044, 6.1382) (8.7636, 6.1207) (8.8216, 6.0996) (8.8508, 6.089) knots 0 0 0 0 0.009192 0.01851 0.01851 0.01851 0.01851
  line L48 (8.8508, 6.089) -> (9.6308, 5.7989)
  line L49 (9.6308, 5.7989) -> (9.6308, 5.6539)
  line L50 (9.6308, 5.6539) -> (8.5571, 6.0743)
  line L51 (8.5571, 6.0743) -> (8.5571, 6.2201)
extrude "Extrude12" cut sketch "Sketch25" against normal blind 0.05 bodies 16
copy_body "Body->Comp1" bodies 17 removing the originals makes body 18 in component "Component"
copy_body "Body->Comp2" bodies 16 removing the originals makes body 19 in component "Component'"
sketch "Sketch26" plane through (0, 1, 0) normal (0, 1, 0) x (-1, 0, 0)
  circle A0 centre (-18.5529, -19.2949) radius 1.8
  circle A1 centre (18.6014, -19.35) radius 1.8
  circle A2 centre (-18.5859, 18.5894) radius 1.8
  circle A3 centre (18.5683, 18.5343) radius 1.8
  line L0 (-21.58, 21.58) -> (-21.58, -21.58)
  line L1 (-21.58, -21.58) -> (21.58, -21.58)
  line L2 (21.58, -21.58) -> (21.58, 21.58)
  line L3 (21.58, 21.58) -> (-21.58, 21.58)
  line L4 (12.1824, 13.4289) -> (1.0281, 13.4289)
  line L5 (1.0281, 13.4289) -> (1.0281, 21.2643)
  line L6 (1.0281, 21.2643) -> (12.1824, 21.2643)
  line L7 (12.1824, 21.2643) -> (12.1824, 13.4289)
extrude "Extrude13" add sketch "Sketch26" along normal blind 10 separate body contours L4 L5 L6 L7 makes body 20
chamfer "Chamfer3" distance 2 angle 45 1 edges at (-6.6052, 11, 21.2643) on bodies 20
chamfer "Chamfer4" distance 2 angle 45 1 edges at (-6.6052, 11, 13.4289) on bodies 20
sketch "Sketch27" plane through (0, 11, 0) normal (0, 1, 0) x (-1, 0, 0)
  line L0 (1.0281, 15.4289) -> (12.1824, 15.4289)
  line L1 (12.1824, 15.4289) -> (12.1824, 19.2643)
  line L2 (12.1824, 19.2643) -> (1.0281, 19.2643)
  line L3 (1.0281, 19.2643) -> (1.0281, 15.4289)
  line L4 (12.1824, 17.3466) -> (1.0281, 17.3466) construction
  circle A0 centre (9.1824, 17.3466) radius 1.5
  circle A1 centre (4.0281, 17.3466) radius 1.5
  line L5 (6.8781, 15.61) -> (6.3781, 15.61)
  line L6 (6.3781, 15.61) -> (6.3781, 18.91)
  line L7 (6.3781, 18.91) -> (6.8781, 18.91)
  line L8 (6.8781, 18.91) -> (6.8781, 15.61)
extrude "Extrude14" cut sketch "Sketch27" against normal blind 2 contours A0 | A1 | L5 L6 L7 L8 bodies 20
sketch "Sketch28" plane through (0, 0, 21.2643) normal (0, 0, 1) x (1, 0, 0)
  line L0 (-1.0281, 9) -> (-12.1824, 9)
  line L1 (-12.1824, 9) -> (-12.1824, 1)
  line L2 (-12.1824, 1) -> (-1.0281, 1)
  line L3 (-1.0281, 1) -> (-1.0281, 9)
  line L4 (-7.6207, 2) -> (-14.2987, 2) construction
  line L5 (-10.1824, 8.5257) -> (-8.5824, 8.5257)
  line L6 (-7.5824, 7.5257) -> (-7.5824, 3)
  line L7 (-8.5824, 2) -> (-10.1824, 2)
  line L8 (-11.1824, 3) -> (-11.1824, 7.5257)
  line L9 (-4.6281, 8.5257) -> (-3.0281, 8.5257)
  line L10 (-2.0281, 7.5257) -> (-2.0281, 3)
  line L11 (-3.0281, 2) -> (-4.6281, 2)
  line L12 (-5.6281, 3) -> (-5.6281, 7.5257)
  arc A0 (-10.1824, 8.5257) -> (-11.1824, 7.5257) centre (-10.1824, 7.5257) ccw
  arc A1 (-7.5824, 7.5257) -> (-8.5824, 8.5257) centre (-8.5824, 7.5257) ccw
  arc A2 (-11.1824, 3) -> (-10.1824, 2) centre (-10.1824, 3) ccw
  arc A3 (-8.5824, 2) -> (-7.5824, 3) centre (-8.5824, 3) ccw
  arc A4 (-4.6281, 8.5257) -> (-5.6281, 7.5257) centre (-4.6281, 7.5257) ccw
  arc A5 (-2.0281, 7.5257) -> (-3.0281, 8.5257) centre (-3.0281, 7.5257) ccw
  arc A6 (-3.0281, 2) -> (-2.0281, 3) centre (-3.0281, 3) ccw
  arc A7 (-5.6281, 3) -> (-4.6281, 2) centre (-4.6281, 3) ccw
  dimension "d133" = 3.6
  dimension "d134" = 3.6
  dimension "d137" = 1
  measures "d137" radius of A0
extrude "Extrude15" cut sketch "Sketch28" against normal blind 2 contours L5 L6 L7 L8 A0 A1 A2 A3 | L9 L10 L11 L12 A4 A5 A6 A7 bodies 20
sketch "Sketch30" plane through (0, 0, 19.2643) normal (0, 0, 1) x (1, 0, 0)
  arc A0 (-11.1824, 3) -> (-10.1824, 2) centre (-10.1824, 3) ccw
  line L0 (-10.1824, 2) -> (-8.5824, 2)
  arc A1 (-8.5824, 2) -> (-7.5824, 3) centre (-8.5824, 3) ccw
  line L1 (-7.5824, 3) -> (-7.5824, 7.5257)
  arc A2 (-7.5824, 7.5257) -> (-8.5824, 8.5257) centre (-8.5824, 7.5257) ccw
  line L2 (-8.5824, 8.5257) -> (-10.1824, 8.5257)
  arc A3 (-10.1824, 8.5257) -> (-11.1824, 7.5257) centre (-10.1824, 7.5257) ccw
  line L3 (-11.1824, 7.5257) -> (-11.1824, 3)
  line L4 (-10.575, 7.7725) -> (-8.1866, 7.7725)
  line L5 (-8.1866, 7.7725) -> (-8.1866, 2.6592)
  line L6 (-8.1866, 2.6592) -> (-10.575, 2.6592)
  line L7 (-10.575, 2.6592) -> (-10.575, 7.7725)
  line L8 (-10.1824, 7.337) -> (-8.5824, 7.337)
  line L9 (-8.5824, 7.337) -> (-8.5824, 3)
  line L10 (-8.5824, 3) -> (-10.1824, 3)
  line L11 (-10.1824, 3) -> (-10.1824, 7.337)
extrude "Extrude16" add sketch "Sketch30" along normal blind 2 separate body contours L4 L5 L6 L7 makes body 21
fillet "Fillet6" radius 0.5 2 edges at (-8.1866, 7.7725, 20.2643) (-8.1866, 2.6592, 20.2643) on bodies 21
fillet "Fillet7" radius 0.5 2 edges at (-10.575, 7.7725, 20.2643) (-10.575, 2.6592, 20.2643) on bodies 21
copy_body "CopyPasteBodies6" bodies 21 makes body 22
move_body "Move6" bodies 22 to x (1, 0, 0) y (0, 1, 0) z (0, 0, 1) at (5.5, 0, 0)
cylinder "CylinderPrimitive4" add diameter 2.643 height 1 placed x (1, 0, 0) y (0, 0, -1) z (0, 1, 0) at (-4.0281, 9, 17.3466) separate body makes body 23
fillet "Fillet8" radius 0.2 1 edges at (-5.2601, 10, 17.8245) on bodies 23
box "BoxPrimitive12" cut length 0.3558 width 1.7789 height -0.2 placed x (0, 0, -1) y (-1, 0, 0) z (0, 1, 0) at (-3.128, 10, 17.5688) bodies 23
copy_body "CopyPasteBodies7" bodies 23 makes body 24
move_body "Move7" bodies 24 to x (1, 0, 0) y (0, 1, 0) z (0, 0, 1) at (-5.15, 0, 0)
copy_body "Body->Comp3" bodies 24 removing the originals makes body 25 in component "Component''"
copy_body "Body->Comp4" bodies 23 removing the originals makes body 26 in component "Component'''"
copy_body "Body->Comp5" bodies 22 removing the originals makes body 27 in component "Component''''"
copy_body "Body->Comp6" bodies 21 removing the originals makes body 28 in component "Component'''''"
copy_body "Body->Comp7" bodies 20 removing the originals makes body 29 in component "Component''''''"
sketch "Sketch35" plane through (0, 1, 0) normal (0, 1, 0) x (-1, 0, 0)
  circle A0 centre (-18.5529, -19.2949) radius 1.8
  circle A1 centre (18.6014, -19.35) radius 1.8
  circle A2 centre (-18.5859, 18.5894) radius 1.8
  circle A3 centre (18.5683, 18.5343) radius 1.8
  line L0 (-21.58, 21.58) -> (-21.58, -21.58)
  line L1 (-21.58, -21.58) -> (21.58, -21.58)
  line L2 (21.58, -21.58) -> (21.58, 21.58)
  line L3 (21.58, 21.58) -> (-21.58, 21.58)
  line L4 (21.58, -16.3408) -> (13.6581, -16.3408)
  line L5 (13.6581, -16.3408) -> (13.6581, -0.2091)
  line L6 (13.6581, -0.2091) -> (21.58, -0.2091)
  line L7 (21.58, -0.2091) -> (21.58, -16.3408)
extrude "Extrude17" add sketch "Sketch35" along normal blind 10 separate body contours L2 L4 L5 L6 L7 makes body 30
chamfer "Chamfer5" distance 1.5 angle 45 2 edges at (-13.6581, 11, -8.2749) (-21.58, 11, -8.2749) on bodies 30
sketch "Sketch36" plane through (0, 11, 0) normal (0, 1, 0) x (-1, 0, 0)
  line L0 (20.08, -16.3408) -> (20.08, -0.2091)
  line L1 (20.08, -0.2091) -> (15.1581, -0.2091)
  line L2 (15.1581, -0.2091) -> (15.1581, -16.3408)
  line L3 (15.1581, -16.3408) -> (20.08, -16.3408)
  line L4 (17.6191, -16.3408) -> (17.6191, -0.2091) construction
  circle A0 centre (17.6191, -13.3408) radius 1.5
  circle A1 centre (17.6191, -8.2749) radius 1.5
  circle A2 centre (17.6191, -3.2091) radius 1.5
  dimension "d161" = 3
  dimension "d162" = 3
  dimension "d163" = 3
  measures "d161" diameter of A0
  measures "d162" diameter of A1
  measures "d163" diameter of A2
extrude "Extrude18" cut sketch "Sketch36" against normal blind 2 contours A0 | A1 | A2 bodies 30
move_face "MoveFace2" by (1, 0, 0) 1 faces at (-3.5831, 9, 17.5377) on bodies 26 in component "Component'''"
box "BoxPrimitive1'" cut length 1.7833 width 0.3586 height -0.1 placed x (0, 0, -1) y (-1, 0, 0) z (0, 1, 0) at (-3.8156, 10, 18.2882) bodies 26 in component "Component'''"
box "BoxPrimitive1''" cut length 1.7483 width 0.3028 height -0.1 placed x (0, 0, -1) y (-1, 0, 0) z (0, 1, 0) at (-8.9994, 10, 18.2835) bodies 25 in component "Component''"
sketch "Sketch39" plane through (0, 11, 0) normal (0, 1, 0) x (-1, 0, 0)
  circle A0 centre (17.6191, -13.3408) radius 1.5
  circle A1 centre (17.6191, -8.2749) radius 1.5
  circle A2 centre (17.6191, -3.2091) radius 1.5
  line L0 (20.08, -16.3408) -> (20.08, -0.2091)
  line L1 (20.08, -0.2091) -> (15.1581, -0.2091)
  line L2 (15.1581, -0.2091) -> (15.1581, -16.3408)
  line L3 (15.1581, -16.3408) -> (20.08, -16.3408)
  line L4 (19.5921, -6.3706) -> (15.6103, -6.3706)
  line L5 (15.6103, -6.3706) -> (15.6103, -5.5561)
  line L6 (15.6103, -5.5561) -> (19.5921, -5.5561)
  line L7 (19.5921, -5.5561) -> (19.5921, -6.3706)
  line L8 (19.6388, -11.456) -> (15.5569, -11.456)
  line L9 (15.5569, -11.456) -> (15.5569, -10.506)
  line L10 (15.5569, -10.506) -> (19.6388, -10.506)
  line L11 (19.6388, -10.506) -> (19.6388, -11.456)
extrude "Extrude19" cut sketch "Sketch39" against normal blind 2 contours L4 L5 L6 L7 | L8 L9 L10 L11 bodies 30
sketch "Sketch44" plane through (-21.58, 0, 0) normal (-1, 0, 0) x (0, 0, 1)
  line L0 (-0.2091, 9.5) -> (-16.3408, 9.5)
  line L1 (-16.3408, 9.5) -> (-16.3408, 1)
  line L2 (-16.3408, 1) -> (-0.2091, 1)
  line L3 (-0.2091, 1) -> (-0.2091, 9.5)
  line L4 (-13.8408, 7.9044) -> (-12.3628, 7.9044)
  line L5 (-11.3628, 6.9044) -> (-11.3628, 3)
  line L6 (-12.3628, 2) -> (-13.8408, 2)
  line L7 (-14.8408, 3) -> (-14.8408, 6.9044)
  arc A0 (-13.8408, 7.9044) -> (-14.8408, 6.9044) centre (-13.8408, 6.9044) ccw
  arc A1 (-11.3628, 6.9044) -> (-12.3628, 7.9044) centre (-12.3628, 6.9044) ccw
  arc A2 (-12.3628, 2) -> (-11.3628, 3) centre (-12.3628, 3) ccw
  arc A3 (-14.8408, 3) -> (-13.8408, 2) centre (-13.8408, 3) ccw
  line L8 (-9.0191, 7.9044) -> (-7.514, 7.9044)
  line L9 (-6.514, 6.9044) -> (-6.514, 2.9933)
  line L10 (-7.514, 1.9933) -> (-9.0191, 1.9933)
  line L11 (-10.0191, 2.9933) -> (-10.0191, 6.9044)
  arc A4 (-9.0191, 7.9044) -> (-10.0191, 6.9044) centre (-9.0191, 6.9044) ccw
  arc A5 (-6.514, 6.9044) -> (-7.514, 7.9044) centre (-7.514, 6.9044) ccw
  arc A6 (-7.514, 1.9933) -> (-6.514, 2.9933) centre (-7.514, 2.9933) ccw
  arc A7 (-10.0191, 2.9933) -> (-9.0191, 1.9933) centre (-9.0191, 2.9933) ccw
  line L12 (-4.2091, 7.9044) -> (-2.661, 7.9044)
  line L13 (-1.661, 6.9044) -> (-1.661, 2.9986)
  line L14 (-2.661, 1.9986) -> (-4.2091, 1.9986)
  line L15 (-5.2091, 2.9986) -> (-5.2091, 6.9044)
  arc A8 (-4.2091, 7.9044) -> (-5.2091, 6.9044) centre (-4.2091, 6.9044) ccw
  arc A9 (-1.661, 6.9044) -> (-2.661, 7.9044) centre (-2.661, 6.9044) ccw
  arc A10 (-2.661, 1.9986) -> (-1.661, 2.9986) centre (-2.661, 2.9986) ccw
  arc A11 (-5.2091, 2.9986) -> (-4.2091, 1.9986) centre (-4.2091, 2.9986) ccw
  dimension "d211" = 1
  dimension "d214" = 1
  dimension "d217" = 1
  dimension "d218" = 1
  measures "d211" radius of A0
  measures "d214" radius of A4
  measures "d217" radius of A8
  measures "d218" radius of A11
extrude "Extrude22" cut sketch "Sketch44" against normal blind 2 contours L12 L13 L14 L15 A8 A9 A10 A11 bodies 30
extrude "Extrude21" cut sketch "Sketch44" against normal blind 2 contours L8 L9 L10 L11 A4 A5 A6 A7 bodies 30
extrude "Extrude20" cut sketch "Sketch44" against normal blind 2 contours L4 L5 L6 L7 A0 A1 A2 A3 bodies 30
box "BoxPrimitive17" add length 3.9835 width 2.4445 height 1.5 placed x (0, 0, -1) y (-1, 0, 0) z (0, 1, 0) at (3.6177, 1, 19.0857) separate body makes body 31
fillet "Fillet9" radius 0.3 2 edges at (3.6177, 2.5, 17.0939) (1.1732, 2.5, 17.0939) on bodies 31
copy_body "CopyPasteBodies8" bodies 31 makes body 32
move_body "Move8" bodies 32 to x (1, 0, 0) y (0, 1, 0) z (0, 0, 1) at (3.65, 0, 0)
copy_body "CopyPasteBodies9" bodies 32 makes body 33
move_body "Move9" bodies 33 to x (1, 0, 0) y (0, 1, 0) z (0, 0, 1) at (3.7, 0, 0)
copy_body "CopyPasteBodies10" bodies 33 makes body 34
move_body "Move10" bodies 34 to x (1, 0, 0) y (0, 1, 0) z (0, 0, 1) at (3.8, 0, 0)
copy_body "CopyPasteBodies11" bodies 34 makes body 35
move_body "Move11" bodies 35 to x (1, 0, 0) y (0, 1, 0) z (0, 0, 1) at (-0.1, 0, -35.1)
copy_body "CopyPasteBodies12" bodies 35 makes body 36
move_body "Move12" bodies 36 to x (1, 0, 0) y (0, 1, 0) z (0, 0, 1) at (-3.75, 0, 0)
copy_body "CopyPasteBodies13" bodies 35 36 makes body 37 makes body 38
move_body "Move13" bodies 37 38 to x (1, 0, 0) y (0, 1, 0) z (0, 0, 1) at (-7.45, 0, 0)
box "BoxPrimitive19" add length 5.8858 width 5.756 height 1 placed x (0, 0, 1) y (1, 0, 0) z (0, 1, 0) at (-5.3713, 1, 3.4365) separate body makes body 39
fillet "Fillet10" radius 0.4 2 edges at (-0.0481, 1.25, 10.2745) (-4.9818, 1.25, 10.2745) on bodies 9
sketch "Sketch51" plane through (0, 1, 0) normal (0, 1, 0) x (-1, 0, 0)
  line L0 (17.8873, 12.9908) -> (19.3305, 12.9908)
  line L1 (19.8305, 12.4908) -> (19.8305, 10.9595)
  line L2 (19.3305, 10.4595) -> (17.8873, 10.4595)
  line L3 (17.3873, 10.9595) -> (17.3873, 12.4908)
  arc A0 (19.3305, 10.4595) -> (19.8305, 10.9595) centre (19.3305, 10.9595) ccw
  arc A1 (17.3873, 10.9595) -> (17.8873, 10.4595) centre (17.8873, 10.9595) ccw
  arc A2 (17.8873, 12.9908) -> (17.3873, 12.4908) centre (17.8873, 12.4908) ccw
  arc A3 (19.8305, 12.4908) -> (19.3305, 12.9908) centre (19.3305, 12.4908) ccw
  line L4 (15.3569, 2.642) -> (19.3717, 2.642)
  line L5 (19.8717, 2.142) -> (19.8717, 0.6887)
  line L6 (19.3717, 0.1887) -> (15.3569, 0.1887)
  line L7 (14.8569, 0.6887) -> (14.8569, 2.142)
  arc A4 (19.8717, 2.142) -> (19.3717, 2.642) centre (19.3717, 2.142) ccw
  arc A5 (19.3717, 0.1887) -> (19.8717, 0.6887) centre (19.3717, 0.6887) ccw
  arc A6 (14.8569, 0.6887) -> (15.3569, 0.1887) centre (15.3569, 0.6887) ccw
  arc A7 (15.3569, 2.642) -> (14.8569, 2.142) centre (15.3569, 2.142) ccw
  dimension "d243" = 2.4433
  dimension "d244" = 2.5313
  dimension "d245" = 0.5
  dimension "d250" = 0.5
  measures "d245" radius of A0
  measures "d250" radius of A4
extrude "Extrude24" add sketch "Sketch51" along normal blind 9 separate body contours L4 L5 L6 L7 A4 A5 A6 A7 makes body 40
extrude "Extrude23" add sketch "Sketch51" along normal blind 1 separate body contours L0 L1 L2 L3 A0 A1 A2 A3 makes body 41
cylinder "CylinderPrimitive5" add diameter 0.5 height 5 placed x (1, 0, 0) y (0, 0, -1) z (0, 1, 0) at (-19.2623, 2, 11.6383) separate body makes body 42
copy_body "CopyPasteBodies14" bodies 41 42 makes body 43 makes body 44
move_body "Move14" bodies 43 44 to x (1, 0, 0) y (0, 1, 0) z (0, 0, 1) at (0, 0, -2.5)
copy_body "CopyPasteBodies15" bodies 41 42 43 44 makes body 45 makes body 46 makes body 47 makes body 48
move_body "Move15" bodies 45 46 47 48 to x (1, 0, 0) y (0, 1, 0) z (0, 0, 1) at (0, 0, -5)
sketch "Sketch53" plane through (0, 10, 0) normal (0, 1, 0) x (-1, 0, 0)
  arc A0 (19.8717, 2.142) -> (19.3717, 2.642) centre (19.3717, 2.142) ccw
  line L0 (19.3717, 2.642) -> (15.3569, 2.642)
  arc A1 (15.3569, 2.642) -> (14.8569, 2.142) centre (15.3569, 2.142) ccw
  line L1 (14.8569, 2.142) -> (14.8569, 0.6887)
  arc A2 (14.8569, 0.6887) -> (15.3569, 0.1887) centre (15.3569, 0.6887) ccw
  line L2 (15.3569, 0.1887) -> (19.3717, 0.1887)
  arc A3 (19.3717, 0.1887) -> (19.8717, 0.6887) centre (19.3717, 0.6887) ccw
  line L3 (19.8717, 0.6887) -> (19.8717, 2.142)
box "BoxPrimitive21" cut length 1.4533 width 4.0148 height -1 placed x (0, 0, -1) y (-1, 0, 0) z (0, 1, 0) at (-15.3569, 10, 2.142) bodies 40
copy_body "CopyPasteBodies16" bodies 40 makes body 49
move_body "Move16" bodies 49 to x (1, 0, 0) y (0, 1, 0) z (0, 0, 1) at (0, 0, 12.9)
move_body "Move17" bodies 40 to x (1, 0, 0) y (0, 1, 0) z (0, 0, 1) at (0, 0, 0.1)
copy_body "CopyPasteBodies17" bodies 49 makes body 50
move_body "Move18" bodies 50 to x (0, 0, -1) y (0, 1, 0) z (1, 0, 0) at (-24.9604, 0, -28.4829)
cylinder "CylinderPrimitive6" add diameter 2 height 0.1 placed x (1, 0, 0) y (0, 0, -1) z (0, 1, 0) at (3.2068, 1, 8.6803) separate body makes body 51
fillet "Fillet11" radius 0.1 1 edges at (2.2745, 1.1, 9.042) on bodies 51
sketch "Sketch55" plane through (0, 0, 0) normal (0, 0, 1) x (1, 0, 0)
  line L0 (3.4677, 2.2) -> (3.4677, 1)
  line L1 (6.1799, 26) -> (6.1799, 1)
  line L2 (2.3068, 1.1) -> (4.1068, 1.1)
  arc A0 (8.5304, 3.0814) -> (3.6177, 0.6669) centre (7.2632, -0.5455) ccw
pipe "Pipe4" add diameter 0.48 path "Sketch55" along A0 separate body makes body 52
move_body "Move21" bodies 51 to x (1, 0, 0) y (0, 1, 0) z (0, 0, 1) at (0, 0, -7.9)
move_body "Move22" bodies 51 to x (1, 0, 0) y (0, 1, 0) z (0, 0, 1) at (0, 0, 0.2)
move_body "Move23" bodies 52 to x (1, 0, 0) y (0, 1, 0) z (0, 0, 1) at (0, 0, 1)